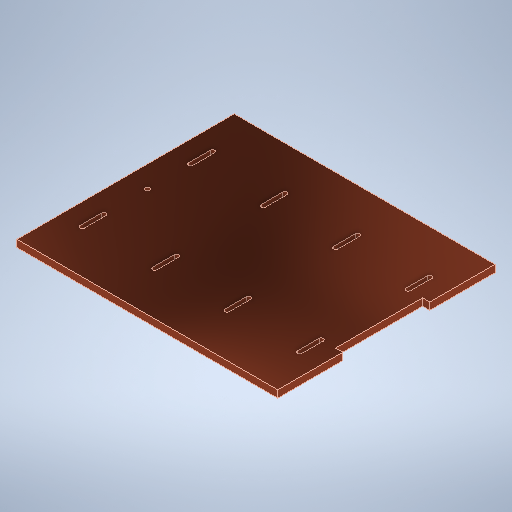
# Autodesk Inventor part: base_2
Saved by Autodesk Inventor 2025.3 (Build 293356030, 356C)
## iProperties
Created: 2026-06-26
Part Number: base_2
Material: Generic
Document SubType Name: Modeling
Designer: user
Density: 1 g/cm^3
Appearance: Copper - Polished
Author: user
Autodesk Inventor part; units mm, degrees
ref_plane "YZ Plane" through (0, 0, 0) normal (1, 0, 0) x (0, 1, 0)
ref_plane "XZ Plane" through (0, 0, 0) normal (0, 1, 0) x (-1, 0, 0)
ref_plane "XY Plane" through (0, 0, 0) normal (0, 0, 1) x (1, 0, 0)
sketch "Sketch1" plane through (0, 0, 0) normal (0, 1, 0) x (-1, 0, 0)
  line L0 (0, 0) -> (-180, 0)
  line L1 (-180, 0) -> (-180, -150)
  line L2 (-180, -150) -> (0, -150)
  line L3 (105, -75) -> (-180, -75) construction
  line L4 (-90, 0) -> (-90, -150) construction
  line L5 (-40, 0) -> (-40, -150) construction
  line L6 (-103, 0) -> (-103, -150) construction
  line L7 (-15, -120) -> (-15, -105) construction
  line L8 (-15, -120) -> (-15, -105) construction
  line L9 (-13.5, -120) -> (-13.5, -105)
  line L10 (-16.5, -105) -> (-16.5, -120)
  arc A0 (-16.5, -120) -> (-13.5, -120) centre (-15, -120) ccw
  arc A1 (-13.5, -105) -> (-16.5, -105) centre (-15, -105) ccw
  line L11 (-65, -120) -> (-65, -105) construction
  line L12 (-65, -120) -> (-65, -105) construction
  line L13 (-66.5, -120) -> (-66.5, -105)
  line L14 (-63.5, -105) -> (-63.5, -120)
  arc A2 (-66.5, -120) -> (-63.5, -120) centre (-65, -120) ccw
  arc A3 (-63.5, -105) -> (-66.5, -105) centre (-65, -105) ccw
  line L15 (-110, -150) -> (-70, -150)
  line L16 (-70, -150) -> (-70, -145)
  line L17 (-70, -145) -> (-110, -145)
  line L18 (-110, -145) -> (-110, -150)
  line L19 (-165, -120) -> (-165, -105) construction
  line L20 (-165, -120) -> (-165, -105) construction
  line L21 (-166.5, -120) -> (-166.5, -105)
  line L22 (-163.5, -105) -> (-163.5, -120)
  arc A4 (-166.5, -120) -> (-163.5, -120) centre (-165, -120) ccw
  arc A5 (-163.5, -105) -> (-166.5, -105) centre (-165, -105) ccw
  line L23 (-116.5, -105) -> (-116.5, -120)
  line L24 (-115, -120) -> (-115, -105) construction
  line L25 (-113.5, -120) -> (-113.5, -105)
  arc A6 (-116.5, -120) -> (-113.5, -120) centre (-115, -120) ccw
  line L26 (-115, -120) -> (-115, -105) construction
  arc A7 (-113.5, -105) -> (-116.5, -105) centre (-115, -105) ccw
  line L27 (-90, -150) -> (-90, 0) construction
  line L28 (-15, -30) -> (-15, -45) construction
  line L29 (-15, -30) -> (-15, -45) construction
  line L30 (-13.5, -30) -> (-13.5, -45)
  line L31 (-16.5, -45) -> (-16.5, -30)
  arc A8 (-13.5, -30) -> (-16.5, -30) centre (-15, -30) ccw
  arc A9 (-16.5, -45) -> (-13.5, -45) centre (-15, -45) ccw
  line L32 (-63.5, -45) -> (-63.5, -30)
  line L33 (-65, -30) -> (-65, -45) construction
  line L34 (-66.5, -30) -> (-66.5, -45)
  arc A10 (-63.5, -30) -> (-66.5, -30) centre (-65, -30) ccw
  line L35 (-65, -30) -> (-65, -45) construction
  arc A11 (-66.5, -45) -> (-63.5, -45) centre (-65, -45) ccw
  line L36 (-110, 0) -> (-70, 0)
  line L37 (-70, 0) -> (-70, -5)
  line L38 (-70, -5) -> (-110, -5)
  line L39 (-110, -5) -> (-110, 0)
  arc A12 (-163.5, -30) -> (-166.5, -30) centre (-165, -30) ccw
  line L40 (-163.5, -45) -> (-163.5, -30)
  line L41 (-165, -30) -> (-165, -45) construction
  line L42 (-165, -30) -> (-165, -45) construction
  arc A13 (-166.5, -45) -> (-163.5, -45) centre (-165, -45) ccw
  line L43 (-166.5, -30) -> (-166.5, -45)
  line L44 (-116.5, -45) -> (-116.5, -30)
  line L45 (-115, -30) -> (-115, -45) construction
  line L46 (-115, -30) -> (-115, -45) construction
  arc A14 (-116.5, -45) -> (-113.5, -45) centre (-115, -45) ccw
  line L47 (-113.5, -30) -> (-113.5, -45)
  arc A15 (-113.5, -30) -> (-116.5, -30) centre (-115, -30) ccw
  line L48 (-180, -2.5) -> (-180, -52.5)
  line L49 (-180, -52.5) -> (-180, -105)
  line L50 (-180, -105) -> (-175, -105)
  line L51 (-175, -105) -> (-175, -45)
  line L52 (-175, -45) -> (-180, -45)
  line L53 (-180, -45) -> (-180, -2.5)
  line L54 (0, -150) -> (0, 0)
  point P0 (-15, -112.5)
  point P1 (-65, -112.5)
  point P2 (-165, -112.5)
  point P3 (-115, -112.5)
  point P4 (-15, -37.5)
  point P5 (-65, -37.5)
  point P6 (-165, -37.5)
  point P7 (-115, -37.5)
  point P8 (-65, -112.5)
  point P9 (-15, -112.5)
  point P10 (-180, -45)
  point P11 (-110, -150)
  point P12 (-70, -150)
  point P13 (-70, 0)
  point P14 (-110, 0)
  point P15 (-165, -112.5)
  dimension "d2" = 15
  dimension "d4" = 30
  dimension "d6" = 1.5
  dimension "d9" = 40
  dimension "d13" = 0
  dimension "d14" = 5
  dimension "d16" = 20
  dimension "d22" = 5
  dimension "d26" = 30
  dimension "d27" = 30
  dimension "d28" = 0
  dimension "d30" = 150
  dimension "d32" = 50
  dimension "d56" = 15
  dimension "d57" = 180
  constraints: 126 end point, 55 symmetric about line, 32 point on circle, 16 centre point, 7 midpoint, 5 equal length, 5 perpendicular, 5 point on line, 4 tangent, 2 horizontal, 1 vertical, 14 other
  measures "d2" distance of L7.start L7.end
  measures "d4" distance from line of L2 L7.start
  measures "d6" radius of A0
  measures "d9" distance of L17.end L16.end
  measures "d13" distance between parallel lines of L2 L15
  measures "d14" distance between parallel lines of L17 L15
  measures "d16" distance between parallel lines of L4 L18
  measures "d22" distance between parallel lines of L49 L51
  measures "d26" distance between parallel lines of L3 L52
  measures "d27" distance between parallel lines of L3 L50
  measures "d28" distance between parallel lines of L1 L48
  measures "d30" distance between parallel lines of L0 L2
  measures "d32" distance of point (-65, -112.5) point (-15, -112.5)
  measures "d56" distance from line of L1 point (-165, -112.5)
  measures "d57" distance between parallel lines of L1 L54
extrude "Extrusion1" add sketch "Sketch1" along normal blind 5 contours L54 L2 L16 L17 L18 L1 L50 L51 L52 L0 L39 L38 L37 | L37 L38 L39 L0 | L2 L18 L17 L16
sketch "Sketch4" plane through (0, 5, 0) normal (0, 1, 0) x (1, 0, 0)
  line L0 (0, 0) -> (180, 0) projected
  line L1 (0, 150) -> (0, 0) projected
  point P0 (15, 75)
  dimension "d76" = 75
  dimension "d77" = 15
  measures "d76" distance from line of L0 point (15, 75)
  measures "d77" distance from line of L1 point (15, 75)
hole "Hole3" at (15, 5, -75) direction (0, -1, 0) diameter 3 end through all
body "Solid1"
